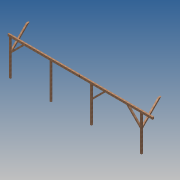
# Autodesk Inventor part: highSide
Saved by Autodesk Inventor 2013 (Build 170138000, 138)
## iProperties
Created: 2013-08-10
Part Number: highSide
Material: Wood (Birch)
Document SubType Name: Modeling
Designer: ddeboer
Mass: 130094 g
Surface Area: 96157.3 cm^2
Volume: 236534 cm^3
Density: 0.55 g/cm^3
Author: ddeboer
Autodesk Inventor part; units mm, degrees
ref_plane "YZ Plane" through (0, 0, 0) normal (1, 0, 0) x (0, 1, 0)
ref_plane "XZ Plane" through (0, 0, 0) normal (0, 1, 0) x (-1, 0, 0)
ref_plane "XY Plane" through (0, 0, 0) normal (0, 0, 1) x (1, 0, 0)
sketch "Sketch1" plane through (0, 0, 0) normal (0, 0, 1) x (1, 0, 0)
  line L0 (0, 0) -> (88.9, 0)
  line L1 (88.9, 0) -> (88.9, 2298.7)
  line L2 (88.9, 2298.7) -> (0, 2298.7)
  line L3 (0, 2298.7) -> (0, 0)
  line L4 (44.45, 2298.7) -> (806.45, 2298.7) construction
  line L5 (806.45, 2298.7) -> (-8566.15, 2298.7)
  line L6 (-8566.15, 2298.7) -> (-8566.15, 2438.4)
  line L7 (-8566.15, 2438.4) -> (806.45, 2438.4)
  line L8 (806.45, 2438.4) -> (806.45, 2298.7)
  line L9 (-3143.25, 0) -> (-3232.15, 0)
  line L10 (-3232.15, 0) -> (-3232.15, 2298.7)
  line L11 (-3232.15, 2298.7) -> (-3143.25, 2298.7)
  line L12 (-3143.25, 2298.7) -> (-3143.25, 0)
  line L13 (-5759.45, 0) -> (-5848.35, 0)
  line L14 (-5848.35, 0) -> (-5848.35, 2298.7)
  line L15 (-5848.35, 2298.7) -> (-5759.45, 2298.7)
  line L16 (-5759.45, 2298.7) -> (-5759.45, 0)
  line L17 (-8382, 0) -> (-8470.9, 0)
  line L18 (-8470.9, 0) -> (-8470.9, 2298.7)
  line L19 (-8470.9, 2298.7) -> (-8382, 2298.7)
  line L20 (-8382, 2298.7) -> (-8382, 0)
  line L21 (0, 1536.7) -> (1081.4669, 1536.7) construction
  line L22 (-3187.7, 2298.7) -> (-3187.7, 0) construction
  line L23 (-3232.15, 1745.1837) -> (-3232.15, 1870.9072)
  line L24 (-4141.2663, 2298.7) -> (-4015.5428, 2298.7)
  line L25 (-3143.25, 1745.1837) -> (-3143.25, 1870.9072)
  line L26 (-2234.1337, 2298.7) -> (-2359.8572, 2298.7)
  line L27 (-8382, 1745.1837) -> (-8382, 1870.9072)
  point P0 (-887.7236, 2298.7)
  point P1 (0, 1766.5764)
  dimension "d0" = 88.9
  dimension "d1" = 2298.7
  dimension "d2" = 762
  dimension "d3" = 9372.6
  dimension "d4" = 139.7
  dimension "d5" = 88.9
  dimension "d6" = 3232.15
  dimension "d7" = 88.9
  dimension "d8" = 2616.2
  dimension "d9" = 88.9
  dimension "d10" = 2622.55
  dimension "d12" = 762
  constraints: 56 end point, 11 point on line, 10 parallel, 6 horizontal, 6 perpendicular, 4 symmetric about line, 3 midpoint, 2 collinear
  measures "d0" distance of L0.start L0.end
  measures "d1" distance of L2.end L0.start
  measures "d2" distance of L4.start L4.end
  measures "d3" distance of L4.end L5.end
  measures "d4" distance of L7.end L4.end
  measures "d5" distance of L9.start L9.end
  measures "d6" distance between parallel lines of L12 L1
  measures "d7" distance of L13.start L13.end
  measures "d8" distance between parallel lines of L16 L12
  measures "d9" distance of L17.start L17.end
  measures "d10" distance between parallel lines of L20 L16
  measures "d12" distance of L2.end L21.start
extrude "Extrusion1" add sketch "Sketch1" along normal blind 88.9
sketch "Sketch4" plane through (0, 0, 88.9) normal (0, 0, 1) x (1, 0, 0)
  line L0 (-3232.15, 2298.7) -> (-3232.15, 0) projected
  line L1 (-3232.15, 0) -> (-3143.25, 0) projected
  line L2 (-3143.25, 0) -> (-3143.25, 2298.7) projected
  line L3 (-3143.25, 2298.7) -> (0, 2298.7) projected
  line L4 (0, 2298.7) -> (0, 0) projected
  line L5 (-8382, 2298.7) -> (-5848.35, 2298.7) projected
  line L6 (-5759.45, 2298.7) -> (-3232.15, 2298.7) projected
  line L7 (0, 1536.7) -> (-762, 2298.7)
  line L8 (0, 1536.7) -> (1437.5812, 1536.7) construction
  line L9 (-887.7236, 2298.7) -> (-28.2137, 1439.1901)
  line L10 (-28.2137, 1439.1901) -> (0, 1410.9764)
  line L11 (0, 1410.9764) -> (0, 1536.7)
  line L12 (-762, 2298.7) -> (-887.7236, 2298.7)
  line L13 (-3232.15, 1536.7) -> (-1794.5688, 1536.7) construction
  line L14 (-3232.15, 1410.9764) -> (-3232.15, 1536.7)
  line L15 (-3994.15, 2298.7) -> (-4119.8736, 2298.7)
  line L16 (-2769.5485, 2298.7) -> (-2769.5485, 1149.35) construction
  line L17 (-7616.4778, 2298.7) -> (-7490.7542, 2298.7)
  line L18 (-7490.7542, 2298.7) -> (-8350.2641, 1439.1901)
  line L19 (-8350.2641, 1439.1901) -> (-8378.4778, 1410.9764)
  line L20 (-8378.4778, 1410.9764) -> (-8378.4778, 1536.7)
  line L21 (-8378.4778, 1536.7) -> (-7616.4778, 2298.7)
  line L22 (-3187.7, 0) -> (-3187.7, 2254.8512) construction
  line L23 (-2381.25, 2298.7) -> (-2255.5264, 2298.7)
  line L24 (-2255.5264, 2298.7) -> (-3115.0363, 1439.1901)
  line L25 (-3115.0363, 1439.1901) -> (-3143.25, 1410.9764)
  line L26 (-3143.25, 1410.9764) -> (-3143.25, 1536.7)
  line L27 (-3143.25, 1536.7) -> (-2381.25, 2298.7)
  dimension "d23" = 135
  dimension "d24" = 762
  constraints: 42 end point, 11 point on line, 4 symmetric about line, 3 collinear, 2 horizontal, 1 midpoint, 1 parallel, 1 perpendicular
  measures "d23" angle of L8 L7
  measures "d24" distance from line of L7.start L3
extrude "Extrusion4" add sketch "Sketch4" against normal blind 88.9 contours L3 L7 L4 L10 L9 | L2 L27 L3 L24 L25 | L5 L18 L19 L20 L21
sketch "Sketch5" plane through (0, 0, 0) normal (0, -1, 0) x (1, 0, 0)
  circle A0 centre (44.45, 44.45) radius 12.7
  dimension "d29" = 25.4
  constraints: 1 centre point
  measures "d29" diameter of A0
extrude "Extrusion5" cut sketch "Sketch5" against normal blind 25.4
sketch "Sketch7" plane through (-8470.9, 0, 0) normal (-1, 0, 0) x (0, 0, 1)
  line L0 (88.9, 2298.7) -> (88.9, 0) projected
  line L1 (0, 2298.7) -> (88.9, 2298.7) projected
  line L2 (0, 2298.7) -> (0, 0) projected
  line L3 (44.45, 2298.7) -> (44.45, 1217.0761) construction
  line L4 (0, 1536.7) -> (-898.0256, 2434.7256)
  line L5 (-960.8874, 2371.8638) -> (-241.618, 1652.5944)
  line L6 (-241.618, 1652.5944) -> (0, 1410.9764)
  line L7 (-960.8874, 2371.8638) -> (-1023.7492, 2434.7256)
  line L8 (0, 1536.7) -> (0, 1410.9764)
  line L9 (-898.0256, 2434.7256) -> (-1007.477, 2544.177)
  line L10 (-1007.477, 2544.177) -> (-1147.9666, 2558.943)
  line L11 (-1023.7492, 2434.7256) -> (-1147.9666, 2558.943)
  point P0 (88.9, 1536.7)
  point P1 (88.9, 1410.9764)
  dimension "d55" = 154.7876
  dimension "d56" = 141
  constraints: 18 end point, 3 parallel, 2 point on line, 2 symmetric about line, 1 midpoint
  measures "d55" distance of L4.end L9.end
  measures "d56" angle of L10 L9
extrude "Extrusion7" add sketch "Sketch7" against normal blind 88.9
sketch "Sketch8" plane through (88.9, 0, 0) normal (1, 0, 0) x (0, 0, -1)
  line L0 (-88.9, 0) -> (-88.9, 2298.7) projected
  line L1 (-88.9, 1540.8372) -> (1181.1, 1540.8372) construction
  line L2 (0, 0) -> (0, 2298.7) projected
  line L3 (0, 2298.7) -> (-88.9, 2298.7) projected
  line L4 (-44.45, 2298.7) -> (-44.45, 1189.3242) construction
  line L5 (0, 1540.8372) -> (898.0256, 2438.8628)
  line L6 (960.8874, 2376.001) -> (34.1715, 1449.2851)
  line L7 (34.1715, 1449.2851) -> (0, 1415.1136)
  line L8 (0, 1540.8372) -> (0, 1415.1136)
  line L9 (960.8874, 2376.001) -> (1023.7492, 2438.8628)
  line L10 (898.0256, 2438.8628) -> (1052.8021, 2593.6393)
  line L11 (1052.8021, 2593.6393) -> (1193.2917, 2608.4053)
  line L12 (1023.7492, 2438.8628) -> (1193.2917, 2608.4053)
  point P0 (-88.9, 1415.1136)
  dimension "d53" = 141
  dimension "d54" = 154.7765
  constraints: 20 end point, 3 parallel, 2 point on line, 2 symmetric about line, 1 horizontal, 1 midpoint
  measures "d53" angle of L10 L11
  measures "d54" horizontal distance of L5.end L10.end
extrude "Extrusion8" add sketch "Sketch8" against normal blind 88.9
sketch "Sketch9" plane through (0, 0, 88.9) normal (0, 0, 1) x (1, 0, 0)
  line L0 (806.45, 2298.7) -> (806.45, 2438.4) projected
  line L1 (806.45, 2438.4) -> (-8566.15, 2438.4) projected
  line L2 (-5759.45, 2298.7) -> (-3232.15, 2298.7) projected
  line L3 (-3949.7, 2438.4) -> (-3949.7, 2298.7) construction
  line L4 (-3968.8785, 2438.4) -> (-3931.1509, 2438.4)
  line L5 (-3931.1509, 2438.4) -> (-3931.1509, 2298.7)
  line L6 (-3931.1509, 2298.7) -> (-3968.8785, 2298.7)
  line L7 (-3968.8785, 2298.7) -> (-3968.8785, 2438.4)
  dimension "d50" = 4756.15
  constraints: 10 end point, 4 point on line, 2 parallel, 2 perpendicular, 1 horizontal
  measures "d50" distance between parallel lines of L0 L3
extrude "Extrusion9" cut sketch "Sketch9" against normal blind 12.7
body "Solid1"
